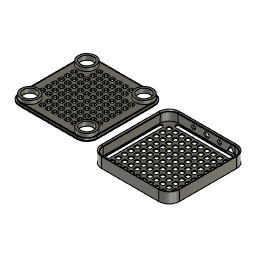
2022_09_10_Foot MidiBox v2 (Autodesk Fusion 360 design; units mm, degrees)
Autodesk Fusion 360 part; units mm, degrees
(part 1 of 3)
sketch "Sketch1" plane through (0, 0, 0) normal (0, 0, 1) x (1, 0, 0)
  line L0 (0, 0) -> (200, 0)
  line L1 (200, 0) -> (200, 200)
  line L2 (200, 200) -> (0, 200)
  line L3 (0, 200) -> (0, 0)
  dimension "d1" = 200
  dimension "d2" = 200
  constraint horizontal L0
  constraint vertical L1
  constraint horizontal L2
  constraint vertical L3
  constraint coincident L0.start L3.end
  measures "d1" distance of L0.start L0.end
  measures "d2" distance of L0.start L2.end
extrude "Extrude1" add sketch "Sketch1" along normal blind 19 makes body 1
sketch "Sketch2" plane through (0, 0, 0) normal (0, 0, 1) x (1, 0, 0)
  circle A0 centre (34.5946, 34.5946) radius 15
  circle A1 centre (34.5946, 34.5946) radius 17
  line L0 (0, 0) -> (200, 0) construction
  line L1 (200, 0) -> (200, 200) construction
  line L2 (200, 200) -> (0, 200) construction
  line L3 (0, 200) -> (0, 0) construction
  line L4 (0, 0) -> (200, 200) construction
  line L5 (200, 0) -> (0, 200) construction
  circle A2 centre (34.5946, 34.5946) radius 20
  line L6 (34.5946, 34.5946) -> (166.2123, 34.5946) construction
  line L7 (166.2123, 34.5946) -> (166.2123, 166.2123) construction
  line L8 (166.2123, 166.2123) -> (34.5946, 166.2123) construction
  line L9 (34.5946, 166.2123) -> (34.5946, 34.5946) construction
  circle A3 centre (166.2123, 34.5946) radius 15
  circle A4 centre (166.2123, 34.5946) radius 17
  circle A5 centre (166.2123, 34.5946) radius 20
  circle A6 centre (166.2123, 166.2123) radius 15
  circle A7 centre (166.2123, 166.2123) radius 17
  circle A8 centre (166.2123, 166.2123) radius 20
  circle A9 centre (34.5946, 166.2123) radius 15
  circle A10 centre (34.5946, 166.2123) radius 17
  circle A11 centre (34.5946, 166.2123) radius 20
  dimension "d5" = 30
  dimension "d6" = 34
  dimension "d7" = 40
  constraint concentric A0 A1
  constraint horizontal L0
  constraint vertical L1
  constraint horizontal L2
  constraint vertical L3
  constraint coincident L0.start L3.end
  constraint perpendicular L4 L5
  constraint coincident A0.centre L4
  constraint concentric A1 A2
  constraint horizontal L6
  constraint vertical L7
  constraint horizontal L8
  constraint vertical L9
  constraint coincident L4 L7.end
  constraint coincident A0.centre A1.centre
  constraint coincident L6.end L7.start
  constraint concentric A3 A5
  constraint coincident L7.end L8.start
  constraint concentric A6 A7
  constraint concentric A7 A8
  constraint coincident L8.end L9.start
  constraint concentric A9 A10
  constraint concentric A10 A11
  constraint equal A2 A11
  constraint equal A2 A8
  constraint equal A2 A5
  constraint equal A1 A4
  constraint equal A1 A7
  constraint equal A1 A10
  constraint equal A0 A9
  constraint equal A0 A3
  constraint equal A0 A6
  measures "d5" diameter of A0
  measures "d6" diameter of A1
  measures "d7" diameter of A2
extrude "Extrude2" add sketch "Sketch2" along normal blind 28 separate body contours A0 | A1 | A2 | A3 | A4 | A5 | A6 | A7 | A8 | A9 | A10 | A11 makes body 2 at (54.4953, 32.6033, 18.6667) makes body 3 at (54.4953, 164.2209, 18.6667) makes body 4 at (186.1129, 164.2209, 18.6667) makes body 5 at (186.1129, 32.6033, 18.6667)
extrude "Extrude3" add sketch "Sketch2" along normal blind 3 separate body contours A0 | A1 | A3 | A4 | A6 | A7 | A9 | A10 makes body 6 at (38.9371, 161.5322, 0) makes body 7 at (166.2123, 45.6438, 0) makes body 8 at (37.0642, 38.5752, 0) makes body 9 at (161.5302, 163.0201, 0)
extrude "Extrude4" add sketch "Sketch2" against normal blind 22.5 contours A0 | A3 | A6 | A9 bodies 6 7 8 9
move_body "Move1" bodies 8 6 7 9 to x (1, 0, 0) y (0, 1, 0) z (0, 0, 1) at (0, 0, 25)
combine "Combine1" operation cut target body 3 tool bodies 6
combine "Combine2" operation cut target body 4 tool bodies 9
combine "Combine3" operation cut target body 5 tool bodies 7
combine "Combine4" operation cut target body 2 tool bodies 8
sketch "Sketch4" plane through (0, 0, 0) normal (0, 0, 1) x (1, 0, 0)
  line L0 (180, 180) -> (22.3709, 180) construction
  line L1 (22.3709, 180) -> (22.3709, 22.3709) construction
  line L2 (22.3709, 22.3709) -> (180, 22.3709) construction
  line L3 (180, 22.3709) -> (180, 180) construction
  line L4 (14.4309, 14.4309) -> (187.94, 14.4309)
  line L5 (187.94, 14.4309) -> (187.94, 187.94)
  line L6 (187.94, 187.94) -> (14.4309, 187.94)
  line L7 (14.4309, 187.94) -> (14.4309, 14.4309)
  line L8 (30.3109, 172.06) -> (30.3109, 30.3109)
  line L9 (30.3109, 30.3109) -> (172.06, 30.3109)
  line L10 (172.06, 30.3109) -> (172.06, 172.06)
  line L11 (172.06, 172.06) -> (30.3109, 172.06)
  line L12 (15.6209, 15.6209) -> (186.75, 15.6209)
  line L13 (186.75, 15.6209) -> (186.75, 186.75)
  line L14 (186.75, 186.75) -> (15.6209, 186.75)
  line L15 (15.6209, 186.75) -> (15.6209, 15.6209)
  line L16 (29.1209, 29.1209) -> (173.25, 29.1209)
  line L17 (173.25, 29.1209) -> (173.25, 173.25)
  line L18 (173.25, 173.25) -> (29.1209, 173.25)
  line L19 (29.1209, 173.25) -> (29.1209, 29.1209)
  dimension "d14" = 7.94
  dimension "d15" = -7.94
  dimension "d16" = 6.75
  dimension "d17" = -6.75
  constraint horizontal L2
  constraint vertical L3
  constraint horizontal L0
  constraint vertical L1
extrude "Extrude5" add sketch "Sketch4" along normal blind 5.25 separate body contours L4 L5 L6 L7 | L12 L13 L14 L15 | L16 L17 L18 L19 makes body 10
sketch "Sketch5" plane through (0, 0, 0) normal (0, 0, 1) x (1, 0, 0)
  line L0 (180, 180) -> (22.3709, 180) construction
  line L1 (22.3709, 180) -> (22.3709, 22.3709) construction
  line L2 (22.3709, 22.3709) -> (180, 22.3709) construction
  line L3 (180, 22.3709) -> (180, 180) construction
  line L4 (166.2123, 34.5946) -> (166.2123, 166.2123) construction
  line L5 (166.2123, 166.2123) -> (34.5946, 166.2123) construction
  line L6 (34.5946, 166.2123) -> (34.5946, 34.5946) construction
  line L7 (34.5946, 34.5946) -> (166.2123, 34.5946) construction
  line L8 (34.5946, 14.5946) -> (166.2123, 14.5946)
  line L9 (186.2123, 34.5946) -> (186.2123, 166.2123)
  line L10 (166.2123, 186.2123) -> (34.5946, 186.2123)
  line L11 (14.5946, 166.2123) -> (14.5946, 34.5946)
  line L12 (166.2123, 186.2123) -> (34.5946, 186.2123)
  line L13 (34.5946, 14.5946) -> (166.2123, 14.5946)
  line L14 (186.2123, 34.5946) -> (186.2123, 166.2123)
  arc A0 (180, 49.0825) -> (150.3825, 22.3709) centre (166.2123, 34.5946) ccw
  arc A1 (186.2123, 166.2123) -> (166.2123, 186.2123) centre (166.2123, 166.2123) ccw
  arc A2 (151.7244, 180) -> (180, 151.7244) centre (166.2123, 166.2123) ccw
  arc A3 (151.7244, 180) -> (180, 151.7244) centre (166.2123, 166.2123) ccw
  arc A4 (186.2123, 166.2123) -> (166.2123, 186.2123) centre (166.2123, 166.2123) ccw
  arc A5 (180, 49.0825) -> (150.3825, 22.3709) centre (166.2123, 34.5946) ccw
  arc A6 (166.2123, 14.5946) -> (186.2123, 34.5946) centre (166.2123, 34.5946) ccw
  arc A7 (50.4244, 22.3709) -> (22.3709, 50.4244) centre (34.5946, 34.5946) ccw
  arc A8 (14.5946, 34.5946) -> (34.5946, 14.5946) centre (34.5946, 34.5946) ccw
  arc A9 (50.4244, 22.3709) -> (22.3709, 50.4244) centre (34.5946, 34.5946) ccw
  arc A10 (14.5946, 34.5946) -> (34.5946, 14.5946) centre (34.5946, 34.5946) ccw
  arc A11 (22.3709, 150.3825) -> (49.0825, 180) centre (34.5946, 166.2123) ccw
  arc A12 (34.5946, 186.2123) -> (14.5946, 166.2123) centre (34.5946, 166.2123) ccw
  arc A13 (22.3709, 150.3825) -> (49.0825, 180) centre (34.5946, 166.2123) ccw
  arc A14 (34.5946, 186.2123) -> (14.5946, 166.2123) centre (34.5946, 166.2123) ccw
  line L15 (187.7123, 34.5946) -> (187.7123, 166.2123)
  arc A15 (187.7123, 166.2123) -> (166.2123, 187.7123) centre (166.2123, 166.2123) ccw
  line L16 (166.2123, 187.7123) -> (34.5946, 187.7123)
  arc A16 (34.5946, 187.7123) -> (13.0946, 166.2123) centre (34.5946, 166.2123) ccw
  line L17 (13.0946, 166.2123) -> (13.0946, 34.5946)
  arc A17 (13.0946, 34.5946) -> (34.5946, 13.0946) centre (34.5946, 34.5946) ccw
  line L18 (34.5946, 13.0946) -> (166.2123, 13.0946)
  arc A18 (166.2123, 13.0946) -> (187.7123, 34.5946) centre (166.2123, 34.5946) ccw
  line L19 (190.2123, 34.5946) -> (190.2123, 166.2123)
  arc A19 (190.2123, 166.2123) -> (166.2123, 190.2123) centre (166.2123, 166.2123) ccw
  line L20 (166.2123, 190.2123) -> (34.5946, 190.2123)
  arc A20 (34.5946, 190.2123) -> (10.5946, 166.2123) centre (34.5946, 166.2123) ccw
  line L21 (10.5946, 166.2123) -> (10.5946, 34.5946)
  arc A21 (10.5946, 34.5946) -> (34.5946, 10.5946) centre (34.5946, 34.5946) ccw
  line L22 (34.5946, 10.5946) -> (166.2123, 10.5946)
  arc A22 (166.2123, 10.5946) -> (190.2123, 34.5946) centre (166.2123, 34.5946) ccw
  dimension "d21" = 40
  dimension "d28" = 40
  dimension "d29" = 1.5
  dimension "d30" = 4
  constraint horizontal L2
  constraint vertical L3
  constraint horizontal L0
  constraint vertical L1
  constraint horizontal L7
  constraint vertical L4
  constraint horizontal L5
  constraint vertical L6
  constraint equal A7 A11
  constraint equal A3 A7
  constraint equal A5 A7
  constraint equal A9 A13
  constraint equal A1 A9
  constraint equal A0 A9
  constraint parallel L7 L8
  constraint parallel L4 L9
  constraint parallel L5 L10
  constraint parallel L6 L11
  constraint coincident L9.end A3
  constraint coincident L10.end A11
  constraint coincident L11.end A7
  constraint coincident L3 A2.end
  constraint coincident L0 A2.start
  constraint concentric A1 A2
  constraint concentric A3 A4
  constraint coincident L3 A0.start
  constraint coincident L2 A0.end
  constraint concentric A5 A6
  constraint coincident L2 A7.start
  constraint coincident L1 A7.end
  constraint concentric A7 A8
  constraint concentric A9 A10
  constraint coincident L1 A11.start
  constraint coincident L0 A11.end
  constraint concentric A11 A12
  constraint concentric A13 A14
  measures "d21" diameter of A7
  measures "d28" diameter of A9
extrude "Extrude7" add sketch "Sketch5" along normal blind 29 separate body contours L8 L9 L10 L11 L12 L13 L14 A1 A4 A6 A8 A10 A12 A14 makes body 11
extrude "Extrude8" cut sketch "Sketch5" along normal blind 10 contours L8 L9 L10 L11 L12 L13 L14 A1 A4 A6 A8 A10 A12 A14 bodies 2 3 4 5
extrude "Extrude10" add sketch "Sketch5" along normal blind 26.5 contours L15 A15 L16 A16 L17 A17 L18 A18 | L19 A19 L20 A20 L21 A21 L22 A22 bodies 11
extrude "Extrude11" add sketch "Sketch5" along normal blind 30 contours L19 A19 L20 A20 L21 A21 L22 A22 bodies 11
extrude "Extrude12" cut 1 faces at (78.4672, 85.1338, 29) along direction (0, 0, -1) blind 27 on bodies 11 bodies 11
extrude "Extrude21" cut 1 faces at (12.2613, 78.4672, 30) along direction (0, 0, -1) blind 5 on bodies 11 bodies 11
extrude "Extrude22" cut 1 faces at (78.4672, 14.0946, 26.5) along direction (0, 0, -1) blind 5 on bodies 11 bodies 11
extrude "Extrude23" cut 1 faces at (12.2613, 78.4672, 25) along direction (0, 0, -1) blind 1 on bodies 11 bodies 11
draft "Draft3" angle 45 neutral plane through (0, 0, 21.5) pull (0, 0, 1) 8 faces at (78.4672, 187.7123, 23.1667) (32.5509, 187.6149, 22.3333) (13.0946, 78.4672, 23.1667) (30.5257, 13.4832, 23.1667) (122.3397, 13.0946, 23.1667) (181.049, 19.0344, 23.1667) (187.7123, 122.3397, 23.1667) (171.2811, 187.1062, 23.1667) on bodies 11
extrude "Extrude24" add sketch "Sketch5" along normal blind 5 separate body contours L8 L9 L10 L11 L12 L13 L14 A1 A4 A6 A8 A10 A12 A14 | L15 A15 L16 A16 L17 A17 L18 A18 | L19 A19 L20 A20 L21 A21 L22 A22 makes body 12
move_body "Move3" bodies 12 to x (1, 0, 0) y (0, 1, 0) z (0, 0, 1) at (0, 0, 23)
move_body "Move4" bodies 3 4 5 2 12 to x (1, 0, 0) y (0, 1, 0) z (0, 0, 1) at (0, 0, -2)
combine "Combine12" operation cut target body 12 tool bodies 11 keep tools
sketch "Sketch8" plane through (0, 0, 0) normal (0, 0, 1) x (1, 0, 0)
sketch "Sketch9" plane through (0, 0, 0) normal (0, 0, 1) x (1, 0, 0)
  line L0 (166.2123, 34.5946) -> (166.2123, 166.2123) construction
  line L1 (166.2123, 166.2123) -> (34.5946, 166.2123) construction
  line L2 (34.5946, 166.2123) -> (34.5946, 34.5946) construction
  line L3 (34.5946, 34.5946) -> (166.2123, 34.5946) construction
  circle A0 centre (34.5946, 166.2123) radius 19
  circle A1 centre (34.5946, 34.5946) radius 19
  circle A2 centre (166.2123, 34.5946) radius 19
  circle A3 centre (166.2123, 166.2123) radius 19
  dimension "d88" = 38
  dimension "d89" = 38
  dimension "d90" = 38
  dimension "d91" = 38
  constraint horizontal L3
  constraint vertical L0
  constraint horizontal L1
  constraint vertical L2
  constraint coincident L1.end L2.start
  constraint coincident L2.end L3.start
  constraint coincident L0.start L3.end
  constraint coincident L0.end L1.start
  measures "d88" diameter of A0
  measures "d89" diameter of A1
  measures "d90" diameter of A2
  measures "d91" diameter of A3
extrude "Extrude25" cut sketch "Sketch9" along normal blind 50 bodies 12
combine "Combine13" operation add target body 12 tool bodies 3 4 5 2
sketch "Sketch10" plane through (0, 186.2123, 0) normal (0, -1, 0) x (1, 0, 0)
  line L0 (166.2123, 21.5) -> (34.5946, 21.5)
  line L1 (34.5946, 21.5) -> (34.5946, 2)
  line L2 (34.5946, 2) -> (166.2123, 2)
  line L3 (166.2123, 2) -> (166.2123, 21.5)
  line L4 (34.5946, 11.75) -> (166.2123, 11.75) construction
  circle A0 centre (100.4035, 11.75) radius 6
  line L5 (100.4035, 11.75) -> (70.4035, 11.75) construction
  circle A1 centre (70.4035, 11.75) radius 4.65
  line L6 (100.4035, 11.75) -> (130, 11.75) construction
  circle A2 centre (130, 11.75) radius 4.65
  line L7 (166.2123, 2) -> (146.2123, 2)
  line L8 (156.2123, 2) -> (156.2123, 18)
  line L9 (146.2123, 2) -> (156.2123, 18)
  line L10 (156.2123, 18) -> (166.2123, 2)
  dimension "d94" = 9.3
  dimension "d95" = 9.3
  dimension "d96" = 30
  dimension "d97" = 12
  dimension "d98" = 20
  dimension "d99" = 16
  constraint midpoint L1 L4.start
  constraint midpoint L3 L4.end
  constraint midpoint L4 A0.centre
  constraint coincident A0.centre L5.start
  constraint coincident L4 L5.end
  constraint parallel L4 L5
  constraint coincident L5.end A1.centre
  constraint coincident L4 L6.end
  constraint parallel L4 L6
  constraint coincident L6.end A2.centre
  constraint coincident L2.end L3.start
  constraint coincident L2 L7.end
  constraint midpoint L7 L8.start
  constraint perpendicular L7 L8
  measures "d94" diameter of A1
  measures "d95" diameter of A2
  measures "d96" distance of A0.centre L5.end
  measures "d97" diameter of A0
  measures "d98" distance of L2.end L7.end
  measures "d99" distance of L8.start L8.end
extrude "Extrude26" cut sketch "Sketch10" against normal blind 55 contours L2 L7 L8 L10 | L2 L7 L8 L9 | A0 | A1 | A2 bodies 11
sketch "Sketch11" plane through (190.2123, 0, 0) normal (1, 0, 0) x (0, 1, 0)
  line L0 (166.2123, 24) -> (34.5946, 24)
  line L1 (34.5946, 24) -> (34.5946, 0)
  line L2 (34.5946, 0) -> (166.2123, 0)
  line L3 (166.2123, 0) -> (166.2123, 24)
  line L4 (34.5946, 0) -> (34.5946, 2)
  line L5 (34.5946, 2) -> (48.5946, 2)
  line L6 (41.5946, 2) -> (41.5946, 19)
  line L7 (34.5946, 2) -> (41.5946, 19)
  line L8 (41.5946, 19) -> (48.5946, 2)
  dimension "d102" = 2
  dimension "d103" = 14
  dimension "d122" = 17
  constraint coincident L1.end L2.start
  constraint vertical L4
  constraint perpendicular L4 L5
  constraint midpoint L5 L6.start
  constraint perpendicular L5 L6
  measures "d102" distance of L1.end L4.end
  measures "d103" distance of L4.end L5.end
  measures "d122" distance of L6.start L6.end
draft "Draft4" angle -3 neutral plane through (0, 0, 21.5) pull (0, 0, 1) 8 faces at (14.5946, 122.3397, 15) (14.6173, 167.1639, 8.5) (44.9809, 186.2123, 11.75) (170.9274, 185.6485, 15) (186.2123, 78.4672, 15) (170.9274, 15.1584, 8.5) (78.4672, 14.5946, 15) (32.6935, 14.6852, 15) on bodies 11
sketch "Sketch12" plane through (0, 0, 2) normal (0, 0, 1) x (-1, 0, 0)
  line L0 (-34.5946, -13.5727) -> (-166.2123, -13.5727)
  arc A0 (-166.2123, -13.5727) -> (-187.2342, -34.5946) centre (-166.2123, -34.5946) ccw
  line L1 (-187.2342, -34.5946) -> (-187.2342, -166.2123)
  arc A1 (-187.2342, -166.2123) -> (-166.2123, -187.2342) centre (-166.2123, -166.2123) ccw
  line L2 (-166.2123, -187.2342) -> (-166.2123, -190.2123)
  line L3 (-166.2123, -190.2123) -> (-146.2123, -190.2123)
  line L4 (-146.2123, -190.2123) -> (-146.2123, -187.2342)
  line L5 (-146.2123, -187.2342) -> (-34.5946, -187.2342)
  arc A2 (-34.5946, -187.2342) -> (-13.5727, -166.2123) centre (-34.5946, -166.2123) ccw
  line L6 (-13.5727, -166.2123) -> (-13.5727, -34.5946)
  arc A3 (-13.5727, -34.5946) -> (-34.5946, -13.5727) centre (-34.5946, -34.5946) ccw
  line L7 (-164.2123, -39.5946) -> (-168.2123, -39.5946)
  line L8 (-171.2123, -36.5946) -> (-171.2123, -32.5946)
  line L9 (-168.2123, -29.5946) -> (-164.2123, -29.5946)
  line L10 (-161.2123, -32.5946) -> (-161.2123, -36.5946)
  line L11 (-161.2123, -39.5946) -> (-171.2123, -29.5946) construction
  line L12 (-171.2123, -39.5946) -> (-161.2123, -29.5946) construction
  arc A4 (-161.2123, -32.5946) -> (-164.2123, -29.5946) centre (-164.2123, -32.5946) ccw
  arc A5 (-168.2123, -29.5946) -> (-171.2123, -32.5946) centre (-168.2123, -32.5946) ccw
  arc A6 (-171.2123, -36.5946) -> (-168.2123, -39.5946) centre (-168.2123, -36.5946) ccw
  arc A7 (-164.2123, -39.5946) -> (-161.2123, -36.5946) centre (-164.2123, -36.5946) ccw
  arc A8 (-146.6011, -32.5946) -> (-149.6011, -29.5946) centre (-149.6011, -32.5946) ccw
  line L13 (-146.6011, -32.5946) -> (-146.6011, -36.5946)
  arc A9 (-149.6011, -39.5946) -> (-146.6011, -36.5946) centre (-149.6011, -36.5946) ccw
  line L14 (-149.6011, -39.5946) -> (-153.6011, -39.5946)
  arc A10 (-156.6011, -36.5946) -> (-153.6011, -39.5946) centre (-153.6011, -36.5946) ccw
  line L15 (-156.6011, -36.5946) -> (-156.6011, -32.5946)
  arc A11 (-153.6011, -29.5946) -> (-156.6011, -32.5946) centre (-153.6011, -32.5946) ccw
  line L16 (-153.6011, -29.5946) -> (-149.6011, -29.5946)
  arc A12 (-131.99, -32.5946) -> (-134.99, -29.5946) centre (-134.99, -32.5946) ccw
  line L17 (-131.99, -32.5946) -> (-131.99, -36.5946)
  arc A13 (-134.99, -39.5946) -> (-131.99, -36.5946) centre (-134.99, -36.5946) ccw
  line L18 (-134.99, -39.5946) -> (-138.99, -39.5946)
  arc A14 (-141.99, -36.5946) -> (-138.99, -39.5946) centre (-138.99, -36.5946) ccw
  line L19 (-141.99, -36.5946) -> (-141.99, -32.5946)
  arc A15 (-138.99, -29.5946) -> (-141.99, -32.5946) centre (-138.99, -32.5946) ccw
  line L20 (-138.99, -29.5946) -> (-134.99, -29.5946)
  arc A16 (-117.3789, -32.5946) -> (-120.3789, -29.5946) centre (-120.3789, -32.5946) ccw
  line L21 (-117.3789, -32.5946) -> (-117.3789, -36.5946)
  arc A17 (-120.3789, -39.5946) -> (-117.3789, -36.5946) centre (-120.3789, -36.5946) ccw
  line L22 (-120.3789, -39.5946) -> (-124.3789, -39.5946)
  arc A18 (-127.3789, -36.5946) -> (-124.3789, -39.5946) centre (-124.3789, -36.5946) ccw
  line L23 (-127.3789, -36.5946) -> (-127.3789, -32.5946)
  arc A19 (-124.3789, -29.5946) -> (-127.3789, -32.5946) centre (-124.3789, -32.5946) ccw
  line L24 (-124.3789, -29.5946) -> (-120.3789, -29.5946)
  arc A20 (-102.7678, -32.5946) -> (-105.7678, -29.5946) centre (-105.7678, -32.5946) ccw
  line L25 (-102.7678, -32.5946) -> (-102.7678, -36.5946)
  arc A21 (-105.7678, -39.5946) -> (-102.7678, -36.5946) centre (-105.7678, -36.5946) ccw
  line L26 (-105.7678, -39.5946) -> (-109.7678, -39.5946)
  arc A22 (-112.7678, -36.5946) -> (-109.7678, -39.5946) centre (-109.7678, -36.5946) ccw
  line L27 (-112.7678, -36.5946) -> (-112.7678, -32.5946)
  arc A23 (-109.7678, -29.5946) -> (-112.7678, -32.5946) centre (-109.7678, -32.5946) ccw
  line L28 (-109.7678, -29.5946) -> (-105.7678, -29.5946)
  arc A24 (-88.1567, -32.5946) -> (-91.1567, -29.5946) centre (-91.1567, -32.5946) ccw
  line L29 (-88.1567, -32.5946) -> (-88.1567, -36.5946)
  arc A25 (-91.1567, -39.5946) -> (-88.1567, -36.5946) centre (-91.1567, -36.5946) ccw
  line L30 (-91.1567, -39.5946) -> (-95.1567, -39.5946)
  arc A26 (-98.1567, -36.5946) -> (-95.1567, -39.5946) centre (-95.1567, -36.5946) ccw
  line L31 (-98.1567, -36.5946) -> (-98.1567, -32.5946)
  arc A27 (-95.1567, -29.5946) -> (-98.1567, -32.5946) centre (-95.1567, -32.5946) ccw
  line L32 (-95.1567, -29.5946) -> (-91.1567, -29.5946)
  arc A28 (-73.5456, -32.5946) -> (-76.5456, -29.5946) centre (-76.5456, -32.5946) ccw
  line L33 (-73.5456, -32.5946) -> (-73.5456, -36.5946)
  arc A29 (-76.5456, -39.5946) -> (-73.5456, -36.5946) centre (-76.5456, -36.5946) ccw
  line L34 (-76.5456, -39.5946) -> (-80.5456, -39.5946)
  arc A30 (-83.5456, -36.5946) -> (-80.5456, -39.5946) centre (-80.5456, -36.5946) ccw
  line L35 (-83.5456, -36.5946) -> (-83.5456, -32.5946)
  arc A31 (-80.5456, -29.5946) -> (-83.5456, -32.5946) centre (-80.5456, -32.5946) ccw
  line L36 (-80.5456, -29.5946) -> (-76.5456, -29.5946)
  arc A32 (-58.9345, -32.5946) -> (-61.9345, -29.5946) centre (-61.9345, -32.5946) ccw
  line L37 (-58.9345, -32.5946) -> (-58.9345, -36.5946)
  arc A33 (-61.9345, -39.5946) -> (-58.9345, -36.5946) centre (-61.9345, -36.5946) ccw
  line L38 (-61.9345, -39.5946) -> (-65.9345, -39.5946)
  arc A34 (-68.9345, -36.5946) -> (-65.9345, -39.5946) centre (-65.9345, -36.5946) ccw
  line L39 (-68.9345, -36.5946) -> (-68.9345, -32.5946)
  arc A35 (-65.9345, -29.5946) -> (-68.9345, -32.5946) centre (-65.9345, -32.5946) ccw
  line L40 (-65.9345, -29.5946) -> (-61.9345, -29.5946)
  arc A36 (-44.3234, -32.5946) -> (-47.3234, -29.5946) centre (-47.3234, -32.5946) ccw
  line L41 (-44.3234, -32.5946) -> (-44.3234, -36.5946)
  arc A37 (-47.3234, -39.5946) -> (-44.3234, -36.5946) centre (-47.3234, -36.5946) ccw
  line L42 (-47.3234, -39.5946) -> (-51.3234, -39.5946)
  arc A38 (-54.3234, -36.5946) -> (-51.3234, -39.5946) centre (-51.3234, -36.5946) ccw
  line L43 (-54.3234, -36.5946) -> (-54.3234, -32.5946)
  arc A39 (-51.3234, -29.5946) -> (-54.3234, -32.5946) centre (-51.3234, -32.5946) ccw
  line L44 (-51.3234, -29.5946) -> (-47.3234, -29.5946)
  arc A40 (-29.7123, -32.5946) -> (-32.7123, -29.5946) centre (-32.7123, -32.5946) ccw
  line L45 (-29.7123, -32.5946) -> (-29.7123, -36.5946)
  arc A41 (-32.7123, -39.5946) -> (-29.7123, -36.5946) centre (-32.7123, -36.5946) ccw
  line L46 (-32.7123, -39.5946) -> (-36.7123, -39.5946)
  arc A42 (-39.7123, -36.5946) -> (-36.7123, -39.5946) centre (-36.7123, -36.5946) ccw
  line L47 (-39.7123, -36.5946) -> (-39.7123, -32.5946)
  arc A43 (-36.7123, -29.5946) -> (-39.7123, -32.5946) centre (-36.7123, -32.5946) ccw
  line L48 (-36.7123, -29.5946) -> (-32.7123, -29.5946)
  arc A44 (-161.2123, -47.2058) -> (-164.2123, -44.2058) centre (-164.2123, -47.2058) ccw
  line L49 (-161.2123, -47.2058) -> (-161.2123, -51.2058)
  arc A45 (-164.2123, -54.2058) -> (-161.2123, -51.2058) centre (-164.2123, -51.2058) ccw
  line L50 (-164.2123, -54.2058) -> (-168.2123, -54.2058)
  arc A46 (-171.2123, -51.2058) -> (-168.2123, -54.2058) centre (-168.2123, -51.2058) ccw
  line L51 (-171.2123, -51.2058) -> (-171.2123, -47.2058)
  arc A47 (-168.2123, -44.2058) -> (-171.2123, -47.2058) centre (-168.2123, -47.2058) ccw
  line L52 (-168.2123, -44.2058) -> (-164.2123, -44.2058)
  arc A48 (-146.6011, -47.2058) -> (-149.6011, -44.2058) centre (-149.6011, -47.2058) ccw
  line L53 (-146.6011, -47.2058) -> (-146.6011, -51.2058)
  arc A49 (-149.6011, -54.2058) -> (-146.6011, -51.2058) centre (-149.6011, -51.2058) ccw
  line L54 (-149.6011, -54.2058) -> (-153.6011, -54.2058)
  arc A50 (-156.6011, -51.2058) -> (-153.6011, -54.2058) centre (-153.6011, -51.2058) ccw
  line L55 (-156.6011, -51.2058) -> (-156.6011, -47.2058)
  arc A51 (-153.6011, -44.2058) -> (-156.6011, -47.2058) centre (-153.6011, -47.2058) ccw
  line L56 (-153.6011, -44.2058) -> (-149.6011, -44.2058)
  arc A52 (-131.99, -47.2058) -> (-134.99, -44.2058) centre (-134.99, -47.2058) ccw
  line L57 (-131.99, -47.2058) -> (-131.99, -51.2058)
  arc A53 (-134.99, -54.2058) -> (-131.99, -51.2058) centre (-134.99, -51.2058) ccw
  line L58 (-134.99, -54.2058) -> (-138.99, -54.2058)
  arc A54 (-141.99, -51.2058) -> (-138.99, -54.2058) centre (-138.99, -51.2058) ccw
  line L59 (-141.99, -51.2058) -> (-141.99, -47.2058)
  arc A55 (-138.99, -44.2058) -> (-141.99, -47.2058) centre (-138.99, -47.2058) ccw
  line L60 (-138.99, -44.2058) -> (-134.99, -44.2058)
  arc A56 (-117.3789, -47.2058) -> (-120.3789, -44.2058) centre (-120.3789, -47.2058) ccw
  line L61 (-117.3789, -47.2058) -> (-117.3789, -51.2058)
  arc A57 (-120.3789, -54.2058) -> (-117.3789, -51.2058) centre (-120.3789, -51.2058) ccw
  line L62 (-120.3789, -54.2058) -> (-124.3789, -54.2058)
  arc A58 (-127.3789, -51.2058) -> (-124.3789, -54.2058) centre (-124.3789, -51.2058) ccw
  line L63 (-127.3789, -51.2058) -> (-127.3789, -47.2058)
  arc A59 (-124.3789, -44.2058) -> (-127.3789, -47.2058) centre (-124.3789, -47.2058) ccw
  line L64 (-124.3789, -44.2058) -> (-120.3789, -44.2058)
  arc A60 (-102.7678, -47.2058) -> (-105.7678, -44.2058) centre (-105.7678, -47.2058) ccw
  line L65 (-102.7678, -47.2058) -> (-102.7678, -51.2058)
  arc A61 (-105.7678, -54.2058) -> (-102.7678, -51.2058) centre (-105.7678, -51.2058) ccw
  line L66 (-105.7678, -54.2058) -> (-109.7678, -54.2058)
  arc A62 (-112.7678, -51.2058) -> (-109.7678, -54.2058) centre (-109.7678, -51.2058) ccw
  line L67 (-112.7678, -51.2058) -> (-112.7678, -47.2058)
  arc A63 (-109.7678, -44.2058) -> (-112.7678, -47.2058) centre (-109.7678, -47.2058) ccw
  line L68 (-109.7678, -44.2058) -> (-105.7678, -44.2058)
  arc A64 (-88.1567, -47.2058) -> (-91.1567, -44.2058) centre (-91.1567, -47.2058) ccw
  line L69 (-88.1567, -47.2058) -> (-88.1567, -51.2058)
  arc A65 (-91.1567, -54.2058) -> (-88.1567, -51.2058) centre (-91.1567, -51.2058) ccw
  line L70 (-91.1567, -54.2058) -> (-95.1567, -54.2058)
  arc A66 (-98.1567, -51.2058) -> (-95.1567, -54.2058) centre (-95.1567, -51.2058) ccw
  line L71 (-98.1567, -51.2058) -> (-98.1567, -47.2058)
  arc A67 (-95.1567, -44.2058) -> (-98.1567, -47.2058) centre (-95.1567, -47.2058) ccw
  line L72 (-95.1567, -44.2058) -> (-91.1567, -44.2058)
  arc A68 (-73.5456, -47.2058) -> (-76.5456, -44.2058) centre (-76.5456, -47.2058) ccw
  line L73 (-73.5456, -47.2058) -> (-73.5456, -51.2058)
  arc A69 (-76.5456, -54.2058) -> (-73.5456, -51.2058) centre (-76.5456, -51.2058) ccw
  line L74 (-76.5456, -54.2058) -> (-80.5456, -54.2058)
  arc A70 (-83.5456, -51.2058) -> (-80.5456, -54.2058) centre (-80.5456, -51.2058) ccw
  line L75 (-83.5456, -51.2058) -> (-83.5456, -47.2058)
  arc A71 (-80.5456, -44.2058) -> (-83.5456, -47.2058) centre (-80.5456, -47.2058) ccw
  line L76 (-80.5456, -44.2058) -> (-76.5456, -44.2058)
  arc A72 (-58.9345, -47.2058) -> (-61.9345, -44.2058) centre (-61.9345, -47.2058) ccw
  line L77 (-58.9345, -47.2058) -> (-58.9345, -51.2058)
  arc A73 (-61.9345, -54.2058) -> (-58.9345, -51.2058) centre (-61.9345, -51.2058) ccw
  line L78 (-61.9345, -54.2058) -> (-65.9345, -54.2058)
  arc A74 (-68.9345, -51.2058) -> (-65.9345, -54.2058) centre (-65.9345, -51.2058) ccw
  line L79 (-68.9345, -51.2058) -> (-68.9345, -47.2058)
  arc A75 (-65.9345, -44.2058) -> (-68.9345, -47.2058) centre (-65.9345, -47.2058) ccw
  line L80 (-65.9345, -44.2058) -> (-61.9345, -44.2058)
  arc A76 (-44.3234, -47.2058) -> (-47.3234, -44.2058) centre (-47.3234, -47.2058) ccw
  line L81 (-44.3234, -47.2058) -> (-44.3234, -51.2058)
  arc A77 (-47.3234, -54.2058) -> (-44.3234, -51.2058) centre (-47.3234, -51.2058) ccw
  line L82 (-47.3234, -54.2058) -> (-51.3234, -54.2058)
  arc A78 (-54.3234, -51.2058) -> (-51.3234, -54.2058) centre (-51.3234, -51.2058) ccw
  line L83 (-54.3234, -51.2058) -> (-54.3234, -47.2058)
  arc A79 (-51.3234, -44.2058) -> (-54.3234, -47.2058) centre (-51.3234, -47.2058) ccw
  line L84 (-51.3234, -44.2058) -> (-47.3234, -44.2058)
  arc A80 (-29.7123, -47.2058) -> (-32.7123, -44.2058) centre (-32.7123, -47.2058) ccw
  line L85 (-29.7123, -47.2058) -> (-29.7123, -51.2058)
  arc A81 (-32.7123, -54.2058) -> (-29.7123, -51.2058) centre (-32.7123, -51.2058) ccw
  line L86 (-32.7123, -54.2058) -> (-36.7123, -54.2058)
  arc A82 (-39.7123, -51.2058) -> (-36.7123, -54.2058) centre (-36.7123, -51.2058) ccw
  line L87 (-39.7123, -51.2058) -> (-39.7123, -47.2058)
  arc A83 (-36.7123, -44.2058) -> (-39.7123, -47.2058) centre (-36.7123, -47.2058) ccw
  line L88 (-36.7123, -44.2058) -> (-32.7123, -44.2058)
  arc A84 (-161.2123, -61.8169) -> (-164.2123, -58.8169) centre (-164.2123, -61.8169) ccw
  line L89 (-161.2123, -61.8169) -> (-161.2123, -65.8169)
  arc A85 (-164.2123, -68.8169) -> (-161.2123, -65.8169) centre (-164.2123, -65.8169) ccw
  line L90 (-164.2123, -68.8169) -> (-168.2123, -68.8169)
  arc A86 (-171.2123, -65.8169) -> (-168.2123, -68.8169) centre (-168.2123, -65.8169) ccw
  line L91 (-171.2123, -65.8169) -> (-171.2123, -61.8169)
  arc A87 (-168.2123, -58.8169) -> (-171.2123, -61.8169) centre (-168.2123, -61.8169) ccw
  line L92 (-168.2123, -58.8169) -> (-164.2123, -58.8169)
  arc A88 (-146.6011, -61.8169) -> (-149.6011, -58.8169) centre (-149.6011, -61.8169) ccw
  line L93 (-146.6011, -61.8169) -> (-146.6011, -65.8169)
  arc A89 (-149.6011, -68.8169) -> (-146.6011, -65.8169) centre (-149.6011, -65.8169) ccw
  line L94 (-149.6011, -68.8169) -> (-153.6011, -68.8169)
  arc A90 (-156.6011, -65.8169) -> (-153.6011, -68.8169) centre (-153.6011, -65.8169) ccw
  line L95 (-156.6011, -65.8169) -> (-156.6011, -61.8169)
  arc A91 (-153.6011, -58.8169) -> (-156.6011, -61.8169) centre (-153.6011, -61.8169) ccw
  line L96 (-153.6011, -58.8169) -> (-149.6011, -58.8169)
  arc A92 (-131.99, -61.8169) -> (-134.99, -58.8169) centre (-134.99, -61.8169) ccw
  line L97 (-131.99, -61.8169) -> (-131.99, -65.8169)
  arc A93 (-134.99, -68.8169) -> (-131.99, -65.8169) centre (-134.99, -65.8169) ccw
  line L98 (-134.99, -68.8169) -> (-138.99, -68.8169)
  arc A94 (-141.99, -65.8169) -> (-138.99, -68.8169) centre (-138.99, -65.8169) ccw
  line L99 (-141.99, -65.8169) -> (-141.99, -61.8169)
  arc A95 (-138.99, -58.8169) -> (-141.99, -61.8169) centre (-138.99, -61.8169) ccw
  line L100 (-138.99, -58.8169) -> (-134.99, -58.8169)
  arc A96 (-117.3789, -61.8169) -> (-120.3789, -58.8169) centre (-120.3789, -61.8169) ccw
  line L101 (-117.3789, -61.8169) -> (-117.3789, -65.8169)
  arc A97 (-120.3789, -68.8169) -> (-117.3789, -65.8169) centre (-120.3789, -65.8169) ccw
  line L102 (-120.3789, -68.8169) -> (-124.3789, -68.8169)
  arc A98 (-127.3789, -65.8169) -> (-124.3789, -68.8169) centre (-124.3789, -65.8169) ccw
  line L103 (-127.3789, -65.8169) -> (-127.3789, -61.8169)
  arc A99 (-124.3789, -58.8169) -> (-127.3789, -61.8169) centre (-124.3789, -61.8169) ccw
  line L104 (-124.3789, -58.8169) -> (-120.3789, -58.8169)
  arc A100 (-102.7678, -61.8169) -> (-105.7678, -58.8169) centre (-105.7678, -61.8169) ccw
  line L105 (-102.7678, -61.8169) -> (-102.7678, -65.8169)
  arc A101 (-105.7678, -68.8169) -> (-102.7678, -65.8169) centre (-105.7678, -65.8169) ccw
  line L106 (-105.7678, -68.8169) -> (-109.7678, -68.8169)
  arc A102 (-112.7678, -65.8169) -> (-109.7678, -68.8169) centre (-109.7678, -65.8169) ccw
  line L107 (-112.7678, -65.8169) -> (-112.7678, -61.8169)
  arc A103 (-109.7678, -58.8169) -> (-112.7678, -61.8169) centre (-109.7678, -61.8169) ccw
  line L108 (-109.7678, -58.8169) -> (-105.7678, -58.8169)
  arc A104 (-88.1567, -61.8169) -> (-91.1567, -58.8169) centre (-91.1567, -61.8169) ccw
  line L109 (-88.1567, -61.8169) -> (-88.1567, -65.8169)
  arc A105 (-91.1567, -68.8169) -> (-88.1567, -65.8169) centre (-91.1567, -65.8169) ccw
  line L110 (-91.1567, -68.8169) -> (-95.1567, -68.8169)
  arc A106 (-98.1567, -65.8169) -> (-95.1567, -68.8169) centre (-95.1567, -65.8169) ccw
  line L111 (-98.1567, -65.8169) -> (-98.1567, -61.8169)
  arc A107 (-95.1567, -58.8169) -> (-98.1567, -61.8169) centre (-95.1567, -61.8169) ccw
  line L112 (-95.1567, -58.8169) -> (-91.1567, -58.8169)
  arc A108 (-73.5456, -61.8169) -> (-76.5456, -58.8169) centre (-76.5456, -61.8169) ccw
  line L113 (-73.5456, -61.8169) -> (-73.5456, -65.8169)
  arc A109 (-76.5456, -68.8169) -> (-73.5456, -65.8169) centre (-76.5456, -65.8169) ccw
  line L114 (-76.5456, -68.8169) -> (-80.5456, -68.8169)
  arc A110 (-83.5456, -65.8169) -> (-80.5456, -68.8169) centre (-80.5456, -65.8169) ccw
  line L115 (-83.5456, -65.8169) -> (-83.5456, -61.8169)
  arc A111 (-80.5456, -58.8169) -> (-83.5456, -61.8169) centre (-80.5456, -61.8169) ccw
  line L116 (-80.5456, -58.8169) -> (-76.5456, -58.8169)
  arc A112 (-58.9345, -61.8169) -> (-61.9345, -58.8169) centre (-61.9345, -61.8169) ccw
  line L117 (-58.9345, -61.8169) -> (-58.9345, -65.8169)
  arc A113 (-61.9345, -68.8169) -> (-58.9345, -65.8169) centre (-61.9345, -65.8169) ccw
  line L118 (-61.9345, -68.8169) -> (-65.9345, -68.8169)
  arc A114 (-68.9345, -65.8169) -> (-65.9345, -68.8169) centre (-65.9345, -65.8169) ccw
  line L119 (-68.9345, -65.8169) -> (-68.9345, -61.8169)
  arc A115 (-65.9345, -58.8169) -> (-68.9345, -61.8169) centre (-65.9345, -61.8169) ccw
  line L120 (-65.9345, -58.8169) -> (-61.9345, -58.8169)
  arc A116 (-44.3234, -61.8169) -> (-47.3234, -58.8169) centre (-47.3234, -61.8169) ccw
  line L121 (-44.3234, -61.8169) -> (-44.3234, -65.8169)
  arc A117 (-47.3234, -68.8169) -> (-44.3234, -65.8169) centre (-47.3234, -65.8169) ccw
  line L122 (-47.3234, -68.8169) -> (-51.3234, -68.8169)
  arc A118 (-54.3234, -65.8169) -> (-51.3234, -68.8169) centre (-51.3234, -65.8169) ccw
  line L123 (-54.3234, -65.8169) -> (-54.3234, -61.8169)
  arc A119 (-51.3234, -58.8169) -> (-54.3234, -61.8169) centre (-51.3234, -61.8169) ccw
  line L124 (-51.3234, -58.8169) -> (-47.3234, -58.8169)
  arc A120 (-29.7123, -61.8169) -> (-32.7123, -58.8169) centre (-32.7123, -61.8169) ccw
  line L125 (-29.7123, -61.8169) -> (-29.7123, -65.8169)
  arc A121 (-32.7123, -68.8169) -> (-29.7123, -65.8169) centre (-32.7123, -65.8169) ccw
  line L126 (-32.7123, -68.8169) -> (-36.7123, -68.8169)
  arc A122 (-39.7123, -65.8169) -> (-36.7123, -68.8169) centre (-36.7123, -65.8169) ccw
  line L127 (-39.7123, -65.8169) -> (-39.7123, -61.8169)
  arc A123 (-36.7123, -58.8169) -> (-39.7123, -61.8169) centre (-36.7123, -61.8169) ccw
  line L128 (-36.7123, -58.8169) -> (-32.7123, -58.8169)
  arc A124 (-161.2123, -76.428) -> (-164.2123, -73.428) centre (-164.2123, -76.428) ccw
  line L129 (-161.2123, -76.428) -> (-161.2123, -80.428)
  arc A125 (-164.2123, -83.428) -> (-161.2123, -80.428) centre (-164.2123, -80.428) ccw
  line L130 (-164.2123, -83.428) -> (-168.2123, -83.428)
  arc A126 (-171.2123, -80.428) -> (-168.2123, -83.428) centre (-168.2123, -80.428) ccw
  line L131 (-171.2123, -80.428) -> (-171.2123, -76.428)
  arc A127 (-168.2123, -73.428) -> (-171.2123, -76.428) centre (-168.2123, -76.428) ccw
  line L132 (-168.2123, -73.428) -> (-164.2123, -73.428)
  arc A128 (-146.6011, -76.428) -> (-149.6011, -73.428) centre (-149.6011, -76.428) ccw
  line L133 (-146.6011, -76.428) -> (-146.6011, -80.428)
  arc A129 (-149.6011, -83.428) -> (-146.6011, -80.428) centre (-149.6011, -80.428) ccw
  line L134 (-149.6011, -83.428) -> (-153.6011, -83.428)
  arc A130 (-156.6011, -80.428) -> (-153.6011, -83.428) centre (-153.6011, -80.428) ccw
  line L135 (-156.6011, -80.428) -> (-156.6011, -76.428)
  arc A131 (-153.6011, -73.428) -> (-156.6011, -76.428) centre (-153.6011, -76.428) ccw
  line L136 (-153.6011, -73.428) -> (-149.6011, -73.428)
  arc A132 (-131.99, -76.428) -> (-134.99, -73.428) centre (-134.99, -76.428) ccw
  line L137 (-131.99, -76.428) -> (-131.99, -80.428)
  arc A133 (-134.99, -83.428) -> (-131.99, -80.428) centre (-134.99, -80.428) ccw
  line L138 (-134.99, -83.428) -> (-138.99, -83.428)
  arc A134 (-141.99, -80.428) -> (-138.99, -83.428) centre (-138.99, -80.428) ccw
  line L139 (-141.99, -80.428) -> (-141.99, -76.428)
  arc A135 (-138.99, -73.428) -> (-141.99, -76.428) centre (-138.99, -76.428) ccw
  line L140 (-138.99, -73.428) -> (-134.99, -73.428)
  arc A136 (-117.3789, -76.428) -> (-120.3789, -73.428) centre (-120.3789, -76.428) ccw
  line L141 (-117.3789, -76.428) -> (-117.3789, -80.428)
  arc A137 (-120.3789, -83.428) -> (-117.3789, -80.428) centre (-120.3789, -80.428) ccw
  line L142 (-120.3789, -83.428) -> (-124.3789, -83.428)
  arc A138 (-127.3789, -80.428) -> (-124.3789, -83.428) centre (-124.3789, -80.428) ccw
  line L143 (-127.3789, -80.428) -> (-127.3789, -76.428)
  arc A139 (-124.3789, -73.428) -> (-127.3789, -76.428) centre (-124.3789, -76.428) ccw
  line L144 (-124.3789, -73.428) -> (-120.3789, -73.428)
  arc A140 (-102.7678, -76.428) -> (-105.7678, -73.428) centre (-105.7678, -76.428) ccw
  line L145 (-102.7678, -76.428) -> (-102.7678, -80.428)
  arc A141 (-105.7678, -83.428) -> (-102.7678, -80.428) centre (-105.7678, -80.428) ccw
  line L146 (-105.7678, -83.428) -> (-109.7678, -83.428)
  arc A142 (-112.7678, -80.428) -> (-109.7678, -83.428) centre (-109.7678, -80.428) ccw
  line L147 (-112.7678, -80.428) -> (-112.7678, -76.428)
  arc A143 (-109.7678, -73.428) -> (-112.7678, -76.428) centre (-109.7678, -76.428) ccw
  line L148 (-109.7678, -73.428) -> (-105.7678, -73.428)
  arc A144 (-88.1567, -76.428) -> (-91.1567, -73.428) centre (-91.1567, -76.428) ccw
  line L149 (-88.1567, -76.428) -> (-88.1567, -80.428)
  arc A145 (-91.1567, -83.428) -> (-88.1567, -80.428) centre (-91.1567, -80.428) ccw
  line L150 (-91.1567, -83.428) -> (-95.1567, -83.428)
  arc A146 (-98.1567, -80.428) -> (-95.1567, -83.428) centre (-95.1567, -80.428) ccw
  line L151 (-98.1567, -80.428) -> (-98.1567, -76.428)
  arc A147 (-95.1567, -73.428) -> (-98.1567, -76.428) centre (-95.1567, -76.428) ccw
  line L152 (-95.1567, -73.428) -> (-91.1567, -73.428)
  arc A148 (-73.5456, -76.428) -> (-76.5456, -73.428) centre (-76.5456, -76.428) ccw
  line L153 (-73.5456, -76.428) -> (-73.5456, -80.428)
  arc A149 (-76.5456, -83.428) -> (-73.5456, -80.428) centre (-76.5456, -80.428) ccw
  line L154 (-76.5456, -83.428) -> (-80.5456, -83.428)
  arc A150 (-83.5456, -80.428) -> (-80.5456, -83.428) centre (-80.5456, -80.428) ccw
  line L155 (-83.5456, -80.428) -> (-83.5456, -76.428)
  arc A151 (-80.5456, -73.428) -> (-83.5456, -76.428) centre (-80.5456, -76.428) ccw
  line L156 (-80.5456, -73.428) -> (-76.5456, -73.428)
  arc A152 (-58.9345, -76.428) -> (-61.9345, -73.428) centre (-61.9345, -76.428) ccw
  line L157 (-58.9345, -76.428) -> (-58.9345, -80.428)
  arc A153 (-61.9345, -83.428) -> (-58.9345, -80.428) centre (-61.9345, -80.428) ccw
  line L158 (-61.9345, -83.428) -> (-65.9345, -83.428)
  arc A154 (-68.9345, -80.428) -> (-65.9345, -83.428) centre (-65.9345, -80.428) ccw
  line L159 (-68.9345, -80.428) -> (-68.9345, -76.428)
  arc A155 (-65.9345, -73.428) -> (-68.9345, -76.428) centre (-65.9345, -76.428) ccw
  line L160 (-65.9345, -73.428) -> (-61.9345, -73.428)
  arc A156 (-44.3234, -76.428) -> (-47.3234, -73.428) centre (-47.3234, -76.428) ccw
  line L161 (-44.3234, -76.428) -> (-44.3234, -80.428)
  arc A157 (-47.3234, -83.428) -> (-44.3234, -80.428) centre (-47.3234, -80.428) ccw
  line L162 (-47.3234, -83.428) -> (-51.3234, -83.428)
  arc A158 (-54.3234, -80.428) -> (-51.3234, -83.428) centre (-51.3234, -80.428) ccw
  line L163 (-54.3234, -80.428) -> (-54.3234, -76.428)
  arc A159 (-51.3234, -73.428) -> (-54.3234, -76.428) centre (-51.3234, -76.428) ccw
  line L164 (-51.3234, -73.428) -> (-47.3234, -73.428)
  arc A160 (-29.7123, -76.428) -> (-32.7123, -73.428) centre (-32.7123, -76.428) ccw
  line L165 (-29.7123, -76.428) -> (-29.7123, -80.428)
  arc A161 (-32.7123, -83.428) -> (-29.7123, -80.428) centre (-32.7123, -80.428) ccw
  line L166 (-32.7123, -83.428) -> (-36.7123, -83.428)
  arc A162 (-39.7123, -80.428) -> (-36.7123, -83.428) centre (-36.7123, -80.428) ccw
  line L167 (-39.7123, -80.428) -> (-39.7123, -76.428)
  arc A163 (-36.7123, -73.428) -> (-39.7123, -76.428) centre (-36.7123, -76.428) ccw
  line L168 (-36.7123, -73.428) -> (-32.7123, -73.428)
  arc A164 (-161.2123, -91.0391) -> (-164.2123, -88.0391) centre (-164.2123, -91.0391) ccw
  line L169 (-161.2123, -91.0391) -> (-161.2123, -95.0391)
  arc A165 (-164.2123, -98.0391) -> (-161.2123, -95.0391) centre (-164.2123, -95.0391) ccw
  line L170 (-164.2123, -98.0391) -> (-168.2123, -98.0391)
  arc A166 (-171.2123, -95.0391) -> (-168.2123, -98.0391) centre (-168.2123, -95.0391) ccw
  line L171 (-171.2123, -95.0391) -> (-171.2123, -91.0391)
  arc A167 (-168.2123, -88.0391) -> (-171.2123, -91.0391) centre (-168.2123, -91.0391) ccw
  line L172 (-168.2123, -88.0391) -> (-164.2123, -88.0391)
  arc A168 (-146.6011, -91.0391) -> (-149.6011, -88.0391) centre (-149.6011, -91.0391) ccw
  line L173 (-146.6011, -91.0391) -> (-146.6011, -95.0391)
  arc A169 (-149.6011, -98.0391) -> (-146.6011, -95.0391) centre (-149.6011, -95.0391) ccw
  line L174 (-149.6011, -98.0391) -> (-153.6011, -98.0391)
  arc A170 (-156.6011, -95.0391) -> (-153.6011, -98.0391) centre (-153.6011, -95.0391) ccw
  line L175 (-156.6011, -95.0391) -> (-156.6011, -91.0391)
  arc A171 (-153.6011, -88.0391) -> (-156.6011, -91.0391) centre (-153.6011, -91.0391) ccw
  line L176 (-153.6011, -88.0391) -> (-149.6011, -88.0391)
  arc A172 (-131.99, -91.0391) -> (-134.99, -88.0391) centre (-134.99, -91.0391) ccw
  line L177 (-131.99, -91.0391) -> (-131.99, -95.0391)
  arc A173 (-134.99, -98.0391) -> (-131.99, -95.0391) centre (-134.99, -95.0391) ccw
  line L178 (-134.99, -98.0391) -> (-138.99, -98.0391)
  arc A174 (-141.99, -95.0391) -> (-138.99, -98.0391) centre (-138.99, -95.0391) ccw
  line L179 (-141.99, -95.0391) -> (-141.99, -91.0391)
  arc A175 (-138.99, -88.0391) -> (-141.99, -91.0391) centre (-138.99, -91.0391) ccw
  line L180 (-138.99, -88.0391) -> (-134.99, -88.0391)
  arc A176 (-117.3789, -91.0391) -> (-120.3789, -88.0391) centre (-120.3789, -91.0391) ccw
  line L181 (-117.3789, -91.0391) -> (-117.3789, -95.0391)
  arc A177 (-120.3789, -98.0391) -> (-117.3789, -95.0391) centre (-120.3789, -95.0391) ccw
  line L182 (-120.3789, -98.0391) -> (-124.3789, -98.0391)
  arc A178 (-127.3789, -95.0391) -> (-124.3789, -98.0391) centre (-124.3789, -95.0391) ccw
  line L183 (-127.3789, -95.0391) -> (-127.3789, -91.0391)
  arc A179 (-124.3789, -88.0391) -> (-127.3789, -91.0391) centre (-124.3789, -91.0391) ccw
  line L184 (-124.3789, -88.0391) -> (-120.3789, -88.0391)
  arc A180 (-102.7678, -91.0391) -> (-105.7678, -88.0391) centre (-105.7678, -91.0391) ccw
  line L185 (-102.7678, -91.0391) -> (-102.7678, -95.0391)
  arc A181 (-105.7678, -98.0391) -> (-102.7678, -95.0391) centre (-105.7678, -95.0391) ccw
  line L186 (-105.7678, -98.0391) -> (-109.7678, -98.0391)
  arc A182 (-112.7678, -95.0391) -> (-109.7678, -98.0391) centre (-109.7678, -95.0391) ccw
  line L187 (-112.7678, -95.0391) -> (-112.7678, -91.0391)
  arc A183 (-109.7678, -88.0391) -> (-112.7678, -91.0391) centre (-109.7678, -91.0391) ccw
  line L188 (-109.7678, -88.0391) -> (-105.7678, -88.0391)
  arc A184 (-88.1567, -91.0391) -> (-91.1567, -88.0391) centre (-91.1567, -91.0391) ccw
  line L189 (-88.1567, -91.0391) -> (-88.1567, -95.0391)
  arc A185 (-91.1567, -98.0391) -> (-88.1567, -95.0391) centre (-91.1567, -95.0391) ccw
  line L190 (-91.1567, -98.0391) -> (-95.1567, -98.0391)
  arc A186 (-98.1567, -95.0391) -> (-95.1567, -98.0391) centre (-95.1567, -95.0391) ccw
  line L191 (-98.1567, -95.0391) -> (-98.1567, -91.0391)
  arc A187 (-95.1567, -88.0391) -> (-98.1567, -91.0391) centre (-95.1567, -91.0391) ccw
  line L192 (-95.1567, -88.0391) -> (-91.1567, -88.0391)
  arc A188 (-73.5456, -91.0391) -> (-76.5456, -88.0391) centre (-76.5456, -91.0391) ccw
  line L193 (-73.5456, -91.0391) -> (-73.5456, -95.0391)
  arc A189 (-76.5456, -98.0391) -> (-73.5456, -95.0391) centre (-76.5456, -95.0391) ccw
  line L194 (-76.5456, -98.0391) -> (-80.5456, -98.0391)
  arc A190 (-83.5456, -95.0391) -> (-80.5456, -98.0391) centre (-80.5456, -95.0391) ccw
  line L195 (-83.5456, -95.0391) -> (-83.5456, -91.0391)
  arc A191 (-80.5456, -88.0391) -> (-83.5456, -91.0391) centre (-80.5456, -91.0391) ccw
  line L196 (-80.5456, -88.0391) -> (-76.5456, -88.0391)
  arc A192 (-58.9345, -91.0391) -> (-61.9345, -88.0391) centre (-61.9345, -91.0391) ccw
  line L197 (-58.9345, -91.0391) -> (-58.9345, -95.0391)
  arc A193 (-61.9345, -98.0391) -> (-58.9345, -95.0391) centre (-61.9345, -95.0391) ccw
  line L198 (-61.9345, -98.0391) -> (-65.9345, -98.0391)
  arc A194 (-68.9345, -95.0391) -> (-65.9345, -98.0391) centre (-65.9345, -95.0391) ccw
  line L199 (-68.9345, -95.0391) -> (-68.9345, -91.0391)
  arc A195 (-65.9345, -88.0391) -> (-68.9345, -91.0391) centre (-65.9345, -91.0391) ccw
  line L200 (-65.9345, -88.0391) -> (-61.9345, -88.0391)
  arc A196 (-44.3234, -91.0391) -> (-47.3234, -88.0391) centre (-47.3234, -91.0391) ccw
  line L201 (-44.3234, -91.0391) -> (-44.3234, -95.0391)
  arc A197 (-47.3234, -98.0391) -> (-44.3234, -95.0391) centre (-47.3234, -95.0391) ccw
  line L202 (-47.3234, -98.0391) -> (-51.3234, -98.0391)
  arc A198 (-54.3234, -95.0391) -> (-51.3234, -98.0391) centre (-51.3234, -95.0391) ccw
  line L203 (-54.3234, -95.0391) -> (-54.3234, -91.0391)
  arc A199 (-51.3234, -88.0391) -> (-54.3234, -91.0391) centre (-51.3234, -91.0391) ccw
  line L204 (-51.3234, -88.0391) -> (-47.3234, -88.0391)
  arc A200 (-29.7123, -91.0391) -> (-32.7123, -88.0391) centre (-32.7123, -91.0391) ccw
  line L205 (-29.7123, -91.0391) -> (-29.7123, -95.0391)
  arc A201 (-32.7123, -98.0391) -> (-29.7123, -95.0391) centre (-32.7123, -95.0391) ccw
  line L206 (-32.7123, -98.0391) -> (-36.7123, -98.0391)
  arc A202 (-39.7123, -95.0391) -> (-36.7123, -98.0391) centre (-36.7123, -95.0391) ccw
  line L207 (-39.7123, -95.0391) -> (-39.7123, -91.0391)
  arc A203 (-36.7123, -88.0391) -> (-39.7123, -91.0391) centre (-36.7123, -91.0391) ccw
  line L208 (-36.7123, -88.0391) -> (-32.7123, -88.0391)
  arc A204 (-161.2123, -105.6502) -> (-164.2123, -102.6502) centre (-164.2123, -105.6502) ccw
  line L209 (-161.2123, -105.6502) -> (-161.2123, -109.6502)
  arc A205 (-164.2123, -112.6502) -> (-161.2123, -109.6502) centre (-164.2123, -109.6502) ccw
  line L210 (-164.2123, -112.6502) -> (-168.2123, -112.6502)
  arc A206 (-171.2123, -109.6502) -> (-168.2123, -112.6502) centre (-168.2123, -109.6502) ccw
  line L211 (-171.2123, -109.6502) -> (-171.2123, -105.6502)
  arc A207 (-168.2123, -102.6502) -> (-171.2123, -105.6502) centre (-168.2123, -105.6502) ccw
  line L212 (-168.2123, -102.6502) -> (-164.2123, -102.6502)
  arc A208 (-146.6011, -105.6502) -> (-149.6011, -102.6502) centre (-149.6011, -105.6502) ccw
  line L213 (-146.6011, -105.6502) -> (-146.6011, -109.6502)
  arc A209 (-149.6011, -112.6502) -> (-146.6011, -109.6502) centre (-149.6011, -109.6502) ccw
  line L214 (-149.6011, -112.6502) -> (-153.6011, -112.6502)
  arc A210 (-156.6011, -109.6502) -> (-153.6011, -112.6502) centre (-153.6011, -109.6502) ccw
  line L215 (-156.6011, -109.6502) -> (-156.6011, -105.6502)
  arc A211 (-153.6011, -102.6502) -> (-156.6011, -105.6502) centre (-153.6011, -105.6502) ccw
  line L216 (-153.6011, -102.6502) -> (-149.6011, -102.6502)
  arc A212 (-131.99, -105.6502) -> (-134.99, -102.6502) centre (-134.99, -105.6502) ccw
  line L217 (-131.99, -105.6502) -> (-131.99, -109.6502)
  arc A213 (-134.99, -112.6502) -> (-131.99, -109.6502) centre (-134.99, -109.6502) ccw
  line L218 (-134.99, -112.6502) -> (-138.99, -112.6502)
  arc A214 (-141.99, -109.6502) -> (-138.99, -112.6502) centre (-138.99, -109.6502) ccw
  line L219 (-141.99, -109.6502) -> (-141.99, -105.6502)
  arc A215 (-138.99, -102.6502) -> (-141.99, -105.6502) centre (-138.99, -105.6502) ccw
  line L220 (-138.99, -102.6502) -> (-134.99, -102.6502)
  arc A216 (-117.3789, -105.6502) -> (-120.3789, -102.6502) centre (-120.3789, -105.6502) ccw
  line L221 (-117.3789, -105.6502) -> (-117.3789, -109.6502)
  arc A217 (-120.3789, -112.6502) -> (-117.3789, -109.6502) centre (-120.3789, -109.6502) ccw
  line L222 (-120.3789, -112.6502) -> (-124.3789, -112.6502)
  arc A218 (-127.3789, -109.6502) -> (-124.3789, -112.6502) centre (-124.3789, -109.6502) ccw
  line L223 (-127.3789, -109.6502) -> (-127.3789, -105.6502)
  arc A219 (-124.3789, -102.6502) -> (-127.3789, -105.6502) centre (-124.3789, -105.6502) ccw
  line L224 (-124.3789, -102.6502) -> (-120.3789, -102.6502)
  arc A220 (-102.7678, -105.6502) -> (-105.7678, -102.6502) centre (-105.7678, -105.6502) ccw
  line L225 (-102.7678, -105.6502) -> (-102.7678, -109.6502)
  arc A221 (-105.7678, -112.6502) -> (-102.7678, -109.6502) centre (-105.7678, -109.6502) ccw
  line L226 (-105.7678, -112.6502) -> (-109.7678, -112.6502)
  arc A222 (-112.7678, -109.6502) -> (-109.7678, -112.6502) centre (-109.7678, -109.6502) ccw
  line L227 (-112.7678, -109.6502) -> (-112.7678, -105.6502)
  arc A223 (-109.7678, -102.6502) -> (-112.7678, -105.6502) centre (-109.7678, -105.6502) ccw
  line L228 (-109.7678, -102.6502) -> (-105.7678, -102.6502)
  arc A224 (-88.1567, -105.6502) -> (-91.1567, -102.6502) centre (-91.1567, -105.6502) ccw
  line L229 (-88.1567, -105.6502) -> (-88.1567, -109.6502)
  arc A225 (-91.1567, -112.6502) -> (-88.1567, -109.6502) centre (-91.1567, -109.6502) ccw
  line L230 (-91.1567, -112.6502) -> (-95.1567, -112.6502)
  arc A226 (-98.1567, -109.6502) -> (-95.1567, -112.6502) centre (-95.1567, -109.6502) ccw
  line L231 (-98.1567, -109.6502) -> (-98.1567, -105.6502)
  arc A227 (-95.1567, -102.6502) -> (-98.1567, -105.6502) centre (-95.1567, -105.6502) ccw
  line L232 (-95.1567, -102.6502) -> (-91.1567, -102.6502)
  arc A228 (-73.5456, -105.6502) -> (-76.5456, -102.6502) centre (-76.5456, -105.6502) ccw
  line L233 (-73.5456, -105.6502) -> (-73.5456, -109.6502)
  arc A229 (-76.5456, -112.6502) -> (-73.5456, -109.6502) centre (-76.5456, -109.6502) ccw
  line L234 (-76.5456, -112.6502) -> (-80.5456, -112.6502)
  arc A230 (-83.5456, -109.6502) -> (-80.5456, -112.6502) centre (-80.5456, -109.6502) ccw
  line L235 (-83.5456, -109.6502) -> (-83.5456, -105.6502)
  arc A231 (-80.5456, -102.6502) -> (-83.5456, -105.6502) centre (-80.5456, -105.6502) ccw